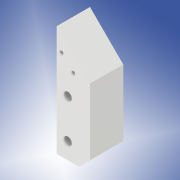
# Autodesk Inventor part: GA005
Saved by Autodesk Inventor 2017 (Build 210142000, 142)
## iProperties
Created: 2017-06-20
Part Number: GA005
Material: ABS Plastic
Document SubType Name: Modeling
Designer: zallen
Density: 1.06 g/cm^3
Appearance: CR White
Author: zallen
Autodesk Inventor part; units mm, degrees
ref_plane "YZ Plane" through (0, 0, 0) normal (1, 0, 0) x (0, 1, 0)
ref_plane "XZ Plane" through (0, 0, 0) normal (0, 1, 0) x (-1, 0, 0)
sketch "Sketch3" plane through (0, 0, 0) normal (0, 0, 1) x (1, 0, 0)
  line L0 (0, 0) -> (0, 100)
  line L1 (0, 0) -> (20, 0)
  line L2 (20, 0) -> (30, 10)
  line L3 (30, 10) -> (30, 70)
  line L4 (30, 70) -> (0, 100)
  circle A0 centre (10, 15) radius 3.6
  circle A1 centre (10, 50) radius 3.6
  point P0 (10, 0)
  dimension "d6" = 100
  dimension "d7" = 20
  dimension "d13" = 10
  dimension "d14" = 10
  dimension "d15" = 7.2
  dimension "d16" = 7.2
  dimension "d17" = 35
  dimension "d18" = 15
  dimension "d33" = 135
  constraints: 10 end point, 2 centre point, 2 vertical alignment, 1 horizontal, 1 midpoint, 1 perpendicular, 1 vertical
  measures "d6" distance of L0.start L0.end
  measures "d7" distance of L0.start L1.end
  measures "d13" horizontal distance of L2.end L1.end
  measures "d14" horizontal distance of L2.end L1.end
  measures "d15" diameter of A0
  measures "d16" diameter of A1
  measures "d17" distance of A0.centre A1.centre
  measures "d18" distance of point (10, 0) A0.centre
  measures "d33" angle of L4 L3
extrude "Extrusion1" add sketch "Sketch3" along normal blind 30
ref_plane "Work Plane1" through (0, 0, 15) normal (0, 0, 1) x (1, 0, 0)
sketch "Sketch4" plane through (0, 0, 15) normal (0, 0, 1) x (1, 0, 0)
  line L0 (0, 100) -> (30, 70) projected
  line L1 (30, 70) -> (30, 10) projected
  line L2 (30, 10) -> (20, 0) projected
  line L3 (20, 0) -> (0, 0) projected
  line L4 (0, 92.9289) -> (25, 67.9289)
  line L5 (25, 67.9289) -> (25, 12.0711)
  line L6 (25, 12.0711) -> (17.9289, 5)
  line L7 (0, 0) -> (0, 100) projected
  line L8 (0, 5) -> (0, 92.9289)
  line L9 (17.9289, 5) -> (17.9289, 0)
  line L10 (17.9289, 0) -> (0, 0)
  line L11 (0, 5) -> (0, 0)
  dimension "d21" = 5
  constraints: 14 end point, 3 point on line, 2 collinear, 2 vertical, 2 other
  measures "d21" distance between parallel lines of L0 L4
extrude "Extrusion2" cut sketch "Sketch4" along normal mid plane 20 contours L4 L5 L6 L9 L3 L7
sketch "Sketch5" plane through (0, 0, 30) normal (0, 0, 1) x (1, 0, 0)
  circle A0 centre (4.3934, 81.4645) radius 1.5
  circle A1 centre (15, 70.8579) radius 1.5
  line L0 (30, 70) -> (0, 100) construction
  line L1 (4.3934, 81.4645) -> (5.8076, 80.0503) construction
  line L2 (5.8076, 80.0503) -> (12.8787, 87.1213) construction
  line L3 (5.8076, 80.0503) -> (15, 70.8579) construction
  point P0 (0, 0)
  point P1 (15, 85)
  dimension "d24" = 3
  dimension "d25" = 3
  dimension "d35" = 2
  dimension "d37" = 13
  dimension "d38" = 10
  constraints: 6 end point, 2 centre point, 1 midpoint, 1 parallel, 1 perpendicular, 1 point on line
  measures "d24" diameter of A0
  measures "d25" diameter of A1
  measures "d35" distance of L1.start L1.end
  measures "d37" distance of L1.end L3.end
  measures "d38" distance from line of L0 L1.start
extrude "Extrusion3" cut sketch "Sketch5" against normal through all
sketch "Sketch7" plane through (0, 0, 5) normal (0, 0, 1) x (1, 0, 0)
  circle A0 centre (10, 50) radius 3.6 projected
  circle A1 centre (10, 15) radius 3.6 projected
  circle A2 centre (10, 50) radius 6.6
  circle A3 centre (10, 15) radius 6.6
  point P0 (0, 0)
  dimension "d45" = 3
  dimension "d46" = 3
  constraints: 2 centre point
  measures "d45" radial gap between concentric circles of A0 A2
  measures "d46" radial gap between concentric circles of A1 A3
extrude "Extrusion5" add sketch "Sketch7" along normal blind 5
sketch "Sketch8" plane through (0, 0, 25) normal (0, 0, -1) x (-1, 0, 0)
  circle A0 centre (-10, 50) radius 3.6 projected
  circle A1 centre (-10, 15) radius 3.6 projected
  circle A2 centre (-10, 50) radius 6.6
  circle A3 centre (-10, 15) radius 6.6
  point P0 (0, 0)
  dimension "d49" = 3
  dimension "d50" = 3
  constraints: 2 centre point
  measures "d49" radial gap between concentric circles of A0 A2
  measures "d50" radial gap between concentric circles of A1 A3
extrude "Extrusion6" add sketch "Sketch8" along normal blind 5
sketch "Sketch9" plane through (0, 0, 5) normal (0, 0, 1) x (1, 0, 0)
  circle A0 centre (4.3934, 81.4645) radius 1.5 projected
  circle A1 centre (15, 70.8579) radius 1.5 projected
  circle A2 centre (4.3934, 81.4645) radius 3.5
  circle A3 centre (15, 70.8579) radius 3.5
  point P0 (0, 0)
  dimension "d53" = 2
  dimension "d54" = 2
  constraints: 2 centre point
  measures "d53" radial gap between concentric circles of A0 A2
  measures "d54" radial gap between concentric circles of A1 A3
extrude "Extrusion7" add sketch "Sketch9" along normal blind 5
sketch "Sketch10" plane through (0, 0, 25) normal (0, 0, -1) x (-1, 0, 0)
  circle A0 centre (-4.3934, 81.4645) radius 1.5 projected
  circle A1 centre (-15, 70.8579) radius 1.5 projected
  circle A2 centre (-4.3934, 81.4645) radius 3.5
  circle A3 centre (-15, 70.8579) radius 3.5
  point P0 (0, 0)
  dimension "d57" = 2
  dimension "d58" = 2
  constraints: 2 centre point
  measures "d57" radial gap between concentric circles of A0 A2
  measures "d58" radial gap between concentric circles of A1 A3
extrude "Extrusion8" add sketch "Sketch10" along normal blind 5
body "Solid1"
